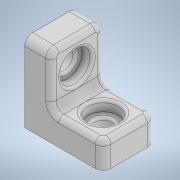
# Autodesk Inventor part: BoardBracketV3
Saved by Autodesk Inventor 2022 (Build 260153000, 153)
## iProperties
Created: 2021-06-18
Part Number: BoardBracketV3
Material: Generic
Document SubType Name: Modeling
Designer: User
Density: 1 g/cm^3
Appearance: Default
Author: User
Autodesk Inventor part; units mm, degrees
ref_plane "YZ Plane" through (0, 0, 0) normal (1, 0, 0) x (0, 1, 0)
ref_plane "XZ Plane" through (0, 0, 0) normal (0, 1, 0) x (-1, 0, 0)
ref_plane "XY Plane" through (0, 0, 0) normal (0, 0, 1) x (1, 0, 0)
sketch "Sketch1" plane through (0, 0, 0) normal (0, 1, 0) x (-1, 0, 0)
  line L0 (5, 5) -> (-5, 5)
  line L1 (-5, 5) -> (-5, -5)
  line L2 (-5, -5) -> (5, -5)
  line L3 (5, -5) -> (5, 5)
  line L4 (5, 5) -> (-5, -5) construction
  line L5 (-5, 5) -> (5, -5) construction
  point P0 (0, 0)
  dimension "d0" = 10
  dimension "d1" = 10
  constraints: 12 end point, 2 midpoint, 2 parallel, 1 horizontal, 1 perpendicular
  measures "d0" distance of L2.end L1.end
  measures "d1" distance of L1.end L0.end
extrude "Extrusion1" add sketch "Sketch1" along normal blind 5
sketch "Sketch2" plane through (0, 0, 0) normal (0, -1, 0) x (1, 0, 0)
  line L0 (-5, -5) -> (-5, 5) projected
  line L1 (-5, 5) -> (-10, 5)
  line L2 (-10, 5) -> (-10, -5)
  line L3 (-10, -5) -> (-5, -5)
  line L4 (-5, -5) -> (-5, 5)
  point P0 (0, 0)
  dimension "d4" = 5
  dimension "d5" = 10
  constraints: 8 end point, 2 parallel, 1 horizontal, 1 perpendicular
  measures "d4" distance of L3.end L2.end
  measures "d5" distance of L2.end L1.end
extrude "Extrusion2" add sketch "Sketch2" against normal blind 15
sketch "Sketch3" plane through (-5, 5, -5) normal (1, 0, 0) x (0, 0, -1)
  line L0 (-10, 0) -> (-10, 10) projected
  line L1 (-10, 0) -> (0, 0) projected
  line L2 (-10, 10) -> (0, 0)
  line L3 (0, 0) -> (-10, 0)
  line L4 (-10, 10) -> (0, 10) projected
  line L5 (-10, 0) -> (0, 10)
  circle A0 centre (-5, 5) radius 3
  point P0 (-5, -5)
  dimension "d8" = 6
  constraints: 6 end point, 1 centre point, 1 collinear, 1 midpoint, 1 perpendicular
  measures "d8" diameter of A0
extrude "Extrusion3" cut sketch "Sketch3" against normal blind 2 contours A0 L2 L5 | L5 L2 A0 | A0 L5 L2 | L2 L5 A0
sketch "Sketch4" plane through (-7, 10, 0) normal (1, 0, 0) x (0, 0, -1)
  circle A0 centre (0, 0) radius 1.75
  point P0 (0, -10)
  dimension "d11" = 3.5
  constraints: 1 centre point
  measures "d11" diameter of A0
extrude "Extrusion4" cut sketch "Sketch4" against normal blind 3
sketch "Sketch5" plane through (0, 5, 0) normal (0, 1, 0) x (1, 0, 0)
  circle A0 centre (0, 0) radius 3
  dimension "d14" = 6
  constraints: 1 centre point, 1 coincident
  measures "d14" diameter of A0
extrude "Extrusion5" cut sketch "Sketch5" against normal blind 2
sketch "Sketch6" plane through (0, 3, 0) normal (0, 1, 0) x (1, 0, 0)
  circle A0 centre (0, 0) radius 3 projected
  circle A1 centre (0, 0) radius 1.75
  dimension "d17" = 3.5
  constraints: 1 centre point, 1 coincident
  measures "d17" diameter of A1
extrude "Extrusion6" cut sketch "Sketch6" against normal blind 3 contours A1
fillet "Fillet1" radius 0.5 4 edges at (-7, 10, 1.75) (-5, 10, 3) (-3, 5, 0) (-1.75, 3, 0)
fillet "Fillet2" radius 1.5 1 edges at (-5, 5, 0)
fillet "Fillet3" radius 1.5 4 edges at (-7.5, 15, 5) (-7.5, 15, -5) (5, 2.5, 5) (5, 2.5, -5)
fillet "Fillet4" radius 1 12 edges at (-5, 14.5607, -4.5607) (-5, 10, -5) (-4.5607, 5.4393, -5) (0, 5, -5) (4.5607, 5, -4.5607) (5, 5, 0) (4.5607, 5, 4.5607) (0, 5, 5) (-4.5607, 5.4393, 5) (-5, 10, 5) (-5, 14.5607, 4.5607) (-5, 15, 0)
body "Solid1"
